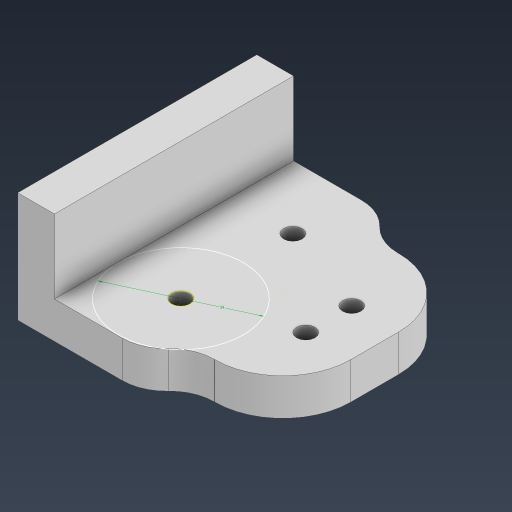
# Autodesk Inventor part: Podstawa
Saved by Autodesk Inventor 2024 (Build 280153000, 153)
## iProperties
Created: 2023-12-19
Part Number: Podstawa
Material: Generic
Document SubType Name: Modeling
Designer: Piter
Density: 1 g/cm^3
Appearance: Default
Author: Piter
Autodesk Inventor part; units mm, degrees
ref_plane "YZ Plane" through (0, 0, 0) normal (1, 0, 0) x (0, 1, 0)
ref_plane "XZ Plane" through (0, 0, 0) normal (0, 1, 0) x (-1, 0, 0)
ref_plane "XY Plane" through (0, 0, 0) normal (0, 0, 1) x (1, 0, 0)
sketch "Sketch1" plane through (0, 0, 0) normal (0, 1, 0) x (-1, 0, 0)
  line L0 (-25, 25) -> (25, 25)
  line L1 (25, 25) -> (25, -25)
  line L2 (25, -25) -> (-25, -25)
  line L3 (-25, -25) -> (-25, 25)
  line L4 (-25, 25) -> (25, -25) construction
  line L5 (25, 25) -> (-25, -25) construction
  line L6 (25, 0) -> (-25, 0)
  circle A0 centre (12.5, 15.25) radius 2.5
  line L7 (-25, 12.5) -> (0, 12.5)
  line L8 (-12.5, 12.5) -> (-12.5, 0)
  circle A1 centre (-12.5, 6.25) radius 2.5
  line L9 (25, -25) -> (-25, 25) construction
  circle A2 centre (12.5, -15.25) radius 2.5
  circle A3 centre (-12.5, -6.25) radius 2.5
  line L10 (0, 32.5) -> (50, 32.5)
  line L11 (50, 32.5) -> (50, -32.5)
  line L12 (50, -32.5) -> (0, -32.5)
  line L13 (0, -32.5) -> (0, 32.5)
  line L14 (0, 32.5) -> (50, -32.5) construction
  line L15 (50, 32.5) -> (0, -32.5) construction
  line L16 (50, -32.5) -> (29.5652, -32.5)
  line L17 (29.5652, -32.5) -> (29.5652, 32.5)
  line L18 (29.5652, 32.5) -> (50, 32.5)
  line L19 (50, 32.5) -> (50, -32.5)
  line L20 (0, 32.5205) -> (0, -32.5)
  circle A4 centre (12.5, -15.25) radius 15
  line L21 (29.5652, -32.5) -> (39.5652, -32.5)
  line L22 (39.5652, -32.5) -> (39.5652, 32.5)
  line L23 (39.5652, 32.5) -> (29.5652, 32.5)
  line L24 (29.5652, 32.5) -> (29.5652, -32.5)
  line L25 (12.5, -15.25) -> (12.5, 0)
  line L26 (-12.5, -6.25) -> (12.5, -6.25)
  point P0 (0, 0)
  point P1 (0, -12.5)
  point P2 (-12.5, -12.5)
  point P3 (0, 25)
  point P4 (0, -25)
  point P5 (0, 25)
  point P6 (0, -25)
  point P7 (0, 32.5)
  point P8 (0, 32.5)
  point P9 (0, -23.5416)
  point P10 (1.101, -25)
  point P11 (25, -23.5416)
  point P12 (23.899, -25)
  point P13 (39.5652, 32.5)
  dimension "d0" = 50
  dimension "d1" = 50
  dimension "d5" = 5
  dimension "d7" = 5
  dimension "d11" = 15.25
  dimension "d12" = 50
  dimension "d13" = 65
  dimension "d19" = 30
  dimension "d21" = 10
  dimension "d27" = 7.5
  dimension "d28" = 7.5
  dimension "d31" = 9
  dimension "d32" = 25
  constraints: 54 end point, 9 parallel, 8 midpoint, 6 perpendicular, 6 point on line, 5 centre point, 4 horizontal, 4 symmetric about line, 1 coincident, 1 vertical, 2 other
  measures "d0" distance of L1.end L2.end
  measures "d1" distance of L0.end L1.end
  measures "d5" diameter of A0
  measures "d7" diameter of A1
  measures "d11" distance from line of A0.centre L6
  measures "d12" distance of L11.end L12.end
  measures "d13" distance of L10.end L11.end
  measures "d19" diameter of A4
  measures "d21" distance of L23.end L22.end
  measures "d27" distance between parallel lines of L2 L12
  measures "d28" distance between parallel lines of L0 L10
  measures "d31" distance from line of L26 A2.centre
  measures "d32" distance of L26.start L26.end
extrude "Extrusion3" add sketch "Sketch1" along normal blind 10 contours L0 L13 L7 L3 | L13 L10 L17 L12 L2 A4 L1 L0 | L0 L1 L6 L13 | L7 L8 A1 L6 L3 | L13 L6 L8 A1 L7 | L6 L13 A4 L2 L3 | L1 A4 L25 L6 | L6 L25 A4 L26 L13 | A4 L1 | L1 A4 L2 L13 L26 L25 | L26 A4 L13 | L13 A4 L2 | L1 L2 A4 | L25 L26 A4 | L13 A4 | L2 A4
extrude "Extrusion4" add sketch "Sketch1" along normal blind 30 contours L10 L22 L12 L17
fillet "Fillet5" radius 12 2 edges at (0, 5, 32.5) (0, 5, -32.5)
fillet "Fillet6" radius 12 2 edges at (0, 5, 25) (0, 5, -25)
fillet "Fillet7" radius 18.5 2 edges at (25, 5, 25) (25, 5, -25)
sketch "Sketch2" plane through (0, 10, 0) normal (0, 1, 0) x (1, 0, 0)
  circle A0 centre (-12.5, -15.25) radius 2.5 projected
  circle A1 centre (-12.5, -15.25) radius 17
  point P0 (0, 0)
  dimension "d34" = 34
  constraints: 1 centre point, 1 coincident
  measures "d34" diameter of A1
body "Solid2"
